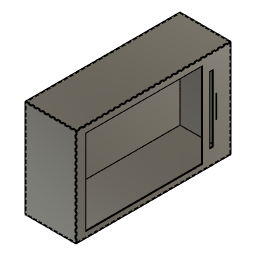
geldautomaat v2 (Autodesk Fusion 360 design; units mm, degrees)
Autodesk Fusion 360 part; units mm, degrees
(part 1 of 3)
sketch "Sketch1" plane through (0, 0, 0) normal (0, 0, 1) x (1, 0, 0)
  line L0 (715.8584, -170.7447) -> (715.8334, -167.7447)
  line L1 (715.8334, -167.7447) -> (707.2277, -167.8174)
  line L2 (707.2277, -167.8174) -> (707.2531, -170.817)
  line L3 (707.2531, -170.817) -> (698.5258, -170.8908)
  line L4 (698.5258, -170.8908) -> (698.5007, -167.8908)
  line L5 (698.5007, -167.8908) -> (689.8951, -167.9631)
  line L6 (689.8951, -167.9631) -> (689.9205, -170.9631)
  line L7 (689.9205, -170.9631) -> (681.1931, -171.0365)
  line L8 (681.1931, -171.0365) -> (681.1677, -168.0365)
  line L9 (681.1677, -168.0365) -> (672.5624, -168.1091)
  line L10 (672.5624, -168.1091) -> (672.5878, -171.1088)
  line L11 (672.5878, -171.1088) -> (663.8601, -171.1825)
  line L12 (663.8601, -171.1825) -> (663.8351, -168.1825)
  line L13 (663.8351, -168.1825) -> (655.2298, -168.2548)
  line L14 (655.2298, -168.2548) -> (655.2552, -171.2548)
  line L15 (655.2552, -171.2548) -> (646.5279, -171.3282)
  line L16 (646.5279, -171.3282) -> (646.5025, -168.3282)
  line L17 (646.5025, -168.3282) -> (637.8972, -168.4005)
  line L18 (637.8972, -168.4005) -> (637.9222, -171.4005)
  line L19 (637.9222, -171.4005) -> (629.1952, -171.4743)
  line L20 (629.1952, -171.4743) -> (629.1702, -168.4743)
  line L21 (629.1702, -168.4743) -> (620.5645, -168.5466)
  line L22 (620.5645, -168.5466) -> (620.5896, -171.5466)
  line L23 (620.5896, -171.5466) -> (611.8626, -171.62)
  line L24 (611.8626, -171.62) -> (611.8372, -168.6199)
  line L25 (611.8372, -168.6199) -> (603.2319, -168.6926)
  line L26 (603.2319, -168.6926) -> (603.257, -171.6923)
  line L27 (603.257, -171.6923) -> (594.5296, -171.7657)
  line L28 (594.5296, -171.7657) -> (594.5046, -168.7664)
  line L29 (594.5046, -168.7664) -> (585.8989, -168.8387)
  line L30 (585.8989, -168.8387) -> (585.9247, -171.8387)
  line L31 (585.9247, -171.8387) -> (577.197, -171.9121)
  line L32 (577.197, -171.9121) -> (577.1719, -168.912)
  line L33 (577.1719, -168.912) -> (568.5663, -168.9844)
  line L34 (568.5663, -168.9844) -> (568.5917, -171.9844)
  line L35 (568.5917, -171.9844) -> (559.8643, -172.0578)
  line L36 (559.8643, -172.0578) -> (559.8389, -169.0581)
  line L37 (559.8389, -169.0581) -> (551.234, -169.1304)
  line L38 (551.234, -169.1304) -> (551.2591, -172.1304)
  line L39 (551.2591, -172.1304) -> (542.5317, -172.2038)
  line L40 (542.5317, -172.2038) -> (542.5063, -169.2038)
  line L41 (542.5063, -169.2038) -> (533.901, -169.2761)
  line L42 (533.901, -169.2761) -> (533.9264, -172.2761)
  line L43 (533.9264, -172.2761) -> (525.1991, -172.3495)
  line L44 (525.1991, -172.3495) -> (525.174, -169.3498)
  line L45 (525.174, -169.3498) -> (516.5684, -169.4222)
  line L46 (516.5684, -169.4222) -> (516.5934, -172.4222)
  line L47 (516.5934, -172.4222) -> (507.8664, -172.4956)
  line L48 (507.8664, -172.4956) -> (507.8414, -169.4955)
  line L49 (507.8414, -169.4955) -> (499.2358, -169.5679)
  line L50 (499.2358, -169.5679) -> (499.2608, -172.5679)
  line L51 (499.2608, -172.5679) -> (490.5338, -172.6413)
  line L52 (490.5338, -172.6413) -> (490.5084, -169.6412)
  line L53 (490.5084, -169.6412) -> (481.9031, -169.7139)
  line L54 (481.9031, -169.7139) -> (481.9285, -172.7136)
  line L55 (481.9285, -172.7136) -> (473.2008, -172.7873)
  line L56 (473.2008, -172.7873) -> (473.1758, -169.7873)
  line L57 (473.1758, -169.7873) -> (464.5705, -169.8596)
  line L58 (464.5705, -169.8596) -> (464.5959, -172.8596)
  line L59 (464.5959, -172.8596) -> (455.8685, -172.933)
  line L60 (455.8685, -172.933) -> (455.8431, -169.933)
  line L61 (455.8431, -169.933) -> (452.8431, -169.9584)
  line L62 (452.8431, -169.9584) -> (452.7782, -162.2135)
  line L63 (452.7782, -162.2135) -> (455.7779, -162.1881)
  line L64 (455.7779, -162.1881) -> (455.7137, -154.5653)
  line L65 (455.7137, -154.5653) -> (452.714, -154.5907)
  line L66 (452.714, -154.5907) -> (452.6487, -146.8459)
  line L67 (452.6487, -146.8459) -> (455.6484, -146.8205)
  line L68 (455.6484, -146.8205) -> (455.5845, -139.1973)
  line L69 (455.5845, -139.1973) -> (452.5845, -139.2227)
  line L70 (452.5845, -139.2227) -> (452.5193, -131.4778)
  line L71 (452.5193, -131.4778) -> (455.5193, -131.4528)
  line L72 (455.5193, -131.4528) -> (455.4551, -123.8296)
  line L73 (455.4551, -123.8296) -> (452.4554, -123.855)
  line L74 (452.4554, -123.855) -> (452.3898, -116.1102)
  line L75 (452.3898, -116.1102) -> (455.3898, -116.0848)
  line L76 (455.3898, -116.0848) -> (455.3256, -108.4616)
  line L77 (455.3256, -108.4616) -> (452.3259, -108.487)
  line L78 (452.3259, -108.487) -> (452.2607, -100.7421)
  line L79 (452.2607, -100.7421) -> (455.2607, -100.7167)
  line L80 (455.2607, -100.7167) -> (455.1961, -93.0943)
  line L81 (455.1961, -93.0943) -> (452.1965, -93.1193)
  line L82 (452.1965, -93.1193) -> (452.1312, -85.3745)
  line L83 (452.1312, -85.3745) -> (455.1312, -85.3494)
  line L84 (455.1312, -85.3494) -> (455.067, -77.7263)
  line L85 (455.067, -77.7263) -> (452.067, -77.7513)
  line L86 (452.067, -77.7513) -> (452.0021, -70.0065)
  line L87 (452.0021, -70.0065) -> (455.0018, -69.9814)
  line L88 (455.0018, -69.9814) -> (454.9376, -62.3583)
  line L89 (454.9376, -62.3583) -> (451.9379, -62.3837)
  line L90 (451.9379, -62.3837) -> (451.8726, -54.6388)
  line L91 (451.8726, -54.6388) -> (454.8723, -54.6137)
  line L92 (454.8723, -54.6137) -> (454.8084, -46.9906)
  line L93 (454.8084, -46.9906) -> (451.8084, -47.0156)
  line L94 (451.8084, -47.0156) -> (451.7432, -39.2708)
  line L95 (451.7432, -39.2708) -> (454.7432, -39.2457)
  line L96 (454.7432, -39.2457) -> (454.679, -31.6229)
  line L97 (454.679, -31.6229) -> (451.6793, -31.648)
  line L98 (451.6793, -31.648) -> (451.614, -23.9031)
  line L99 (451.614, -23.9031) -> (454.6137, -23.8781)
  line L100 (454.6137, -23.8781) -> (454.5887, -20.878)
  line L101 (454.5887, -20.878) -> (463.316, -20.8047)
  line L102 (463.316, -20.8047) -> (463.3411, -23.8043)
  line L103 (463.3411, -23.8043) -> (471.9467, -23.7317)
  line L104 (471.9467, -23.7317) -> (471.9209, -20.732)
  line L105 (471.9209, -20.732) -> (480.6486, -20.6586)
  line L106 (480.6486, -20.6586) -> (480.6737, -23.6583)
  line L107 (480.6737, -23.6583) -> (489.2793, -23.586)
  line L108 (489.2793, -23.586) -> (489.2539, -20.5859)
  line L109 (489.2539, -20.5859) -> (497.9813, -20.5126)
  line L110 (497.9813, -20.5126) -> (498.0067, -23.5122)
  line L111 (498.0067, -23.5122) -> (506.6116, -23.4399)
  line L112 (506.6116, -23.4399) -> (506.5866, -20.4399)
  line L113 (506.5866, -20.4399) -> (515.3136, -20.3665)
  line L114 (515.3136, -20.3665) -> (515.3393, -23.3665)
  line L115 (515.3393, -23.3665) -> (523.9446, -23.2942)
  line L116 (523.9446, -23.2942) -> (523.9192, -20.2942)
  line L117 (523.9192, -20.2942) -> (532.6465, -20.2208)
  line L118 (532.6465, -20.2208) -> (532.6716, -23.2208)
  line L119 (532.6716, -23.2208) -> (541.2772, -23.1482)
  line L120 (541.2772, -23.1482) -> (541.2518, -20.1481)
  line L121 (541.2518, -20.1481) -> (549.9792, -20.0748)
  line L122 (549.9792, -20.0748) -> (550.0042, -23.0748)
  line L123 (550.0042, -23.0748) -> (558.6099, -23.0025)
  line L124 (558.6099, -23.0025) -> (558.5848, -20.0024)
  line L125 (558.5848, -20.0024) -> (567.3118, -19.9291)
  line L126 (567.3118, -19.9291) -> (567.3372, -22.9291)
  line L127 (567.3372, -22.9291) -> (575.9425, -22.8564)
  line L128 (575.9425, -22.8564) -> (575.9171, -19.8568)
  line L129 (575.9171, -19.8568) -> (584.6448, -19.783)
  line L130 (584.6448, -19.783) -> (584.6698, -22.783)
  line L131 (584.6698, -22.783) -> (593.2751, -22.7107)
  line L132 (593.2751, -22.7107) -> (593.2497, -19.7107)
  line L133 (593.2497, -19.7107) -> (601.9771, -19.6373)
  line L134 (601.9771, -19.6373) -> (602.0025, -22.6373)
  line L135 (602.0025, -22.6373) -> (610.6078, -22.5647)
  line L136 (610.6078, -22.5647) -> (610.5827, -19.565)
  line L137 (610.5827, -19.565) -> (619.3097, -19.4913)
  line L138 (619.3097, -19.4913) -> (619.3355, -22.4913)
  line L139 (619.3355, -22.4913) -> (627.9404, -22.419)
  line L140 (627.9404, -22.419) -> (627.9154, -19.419)
  line L141 (627.9154, -19.419) -> (636.6424, -19.3456)
  line L142 (636.6424, -19.3456) -> (636.6678, -22.3456)
  line L143 (636.6678, -22.3456) -> (645.2734, -22.2733)
  line L144 (645.2734, -22.2733) -> (645.248, -19.2733)
  line L145 (645.248, -19.2733) -> (653.9753, -19.1995)
  line L146 (653.9753, -19.1995) -> (654.0004, -22.1995)
  line L147 (654.0004, -22.1995) -> (662.606, -22.1272)
  line L148 (662.606, -22.1272) -> (662.5806, -19.1272)
  line L149 (662.5806, -19.1272) -> (671.308, -19.0538)
  line L150 (671.308, -19.0538) -> (671.333, -22.0538)
  line L151 (671.333, -22.0538) -> (679.9387, -21.9815)
  line L152 (679.9387, -21.9815) -> (679.9133, -18.9815)
  line L153 (679.9133, -18.9815) -> (688.6406, -18.9081)
  line L154 (688.6406, -18.9081) -> (688.666, -21.9078)
  line L155 (688.666, -21.9078) -> (697.2709, -21.8355)
  line L156 (697.2709, -21.8355) -> (697.2459, -18.8355)
  line L157 (697.2459, -18.8355) -> (705.9732, -18.7621)
  line L158 (705.9732, -18.7621) -> (705.9986, -21.7621)
  line L159 (705.9986, -21.7621) -> (714.6039, -21.6894)
  line L160 (714.6039, -21.6894) -> (714.5785, -18.6898)
  line L161 (714.5785, -18.6898) -> (723.3059, -18.6164)
  line L162 (723.3059, -18.6164) -> (723.3313, -21.6157)
  line L163 (723.3313, -21.6157) -> (731.9366, -21.5434)
  line L164 (731.9366, -21.5434) -> (731.9115, -18.5434)
  line L165 (731.9115, -18.5434) -> (740.6385, -18.47)
  line L166 (740.6385, -18.47) -> (740.6639, -21.47)
  line L167 (740.6639, -21.47) -> (743.6636, -21.445)
  line L168 (743.6636, -21.445) -> (743.7288, -29.1898)
  line L169 (743.7288, -29.1898) -> (740.7292, -29.2149)
  line L170 (740.7292, -29.2149) -> (740.7934, -36.838)
  line L171 (740.7934, -36.838) -> (743.7934, -36.813)
  line L172 (743.7934, -36.813) -> (743.8583, -44.5578)
  line L173 (743.8583, -44.5578) -> (740.8583, -44.5829)
  line L174 (740.8583, -44.5829) -> (740.9225, -52.2057)
  line L175 (740.9225, -52.2057) -> (743.9225, -52.1806)
  line L176 (743.9225, -52.1806) -> (743.9874, -59.9252)
  line L177 (743.9874, -59.9252) -> (740.9878, -59.9506)
  line L178 (740.9878, -59.9506) -> (741.052, -67.5737)
  line L179 (741.052, -67.5737) -> (744.052, -67.5487)
  line L180 (744.052, -67.5487) -> (744.1169, -75.2935)
  line L181 (744.1169, -75.2935) -> (741.1172, -75.3186)
  line L182 (741.1172, -75.3186) -> (741.1811, -82.9414)
  line L183 (741.1811, -82.9414) -> (744.1811, -82.9163)
  line L184 (744.1811, -82.9163) -> (744.2464, -90.6612)
  line L185 (744.2464, -90.6612) -> (741.2467, -90.6862)
  line L186 (741.2467, -90.6862) -> (741.3106, -98.3094)
  line L187 (741.3106, -98.3094) -> (744.3106, -98.2843)
  line L188 (744.3106, -98.2843) -> (744.3758, -106.0289)
  line L189 (744.3758, -106.0289) -> (741.3758, -106.0543)
  line L190 (741.3758, -106.0543) -> (741.44, -113.6771)
  line L191 (741.44, -113.6771) -> (744.44, -113.6517)
  line L192 (744.44, -113.6517) -> (744.5049, -121.3969)
  line L193 (744.5049, -121.3969) -> (741.5053, -121.4219)
  line L194 (741.5053, -121.4219) -> (741.5695, -129.0451)
  line L195 (741.5695, -129.0451) -> (744.5692, -129.02)
  line L196 (744.5692, -129.02) -> (744.6344, -136.7645)
  line L197 (744.6344, -136.7645) -> (741.6344, -136.7899)
  line L198 (741.6344, -136.7899) -> (741.6986, -144.4128)
  line L199 (741.6986, -144.4128) -> (744.6986, -144.3877)
  line L200 (744.6986, -144.3877) -> (744.7635, -152.1322)
  line L201 (744.7635, -152.1322) -> (741.7639, -152.1576)
  line L202 (741.7639, -152.1576) -> (741.8281, -159.7808)
  line L203 (741.8281, -159.7808) -> (744.8277, -159.7554)
  line L204 (744.8277, -159.7554) -> (744.8934, -167.5002)
  line L205 (744.8934, -167.5002) -> (741.8933, -167.5256)
  line L206 (741.8933, -167.5256) -> (741.9184, -170.5256)
  line L207 (741.9184, -170.5256) -> (733.191, -170.599)
  line L208 (733.191, -170.599) -> (733.166, -167.5987)
  line L209 (733.166, -167.5987) -> (724.5607, -167.6717)
  line L210 (724.5607, -167.6717) -> (724.5858, -170.6713)
  line L211 (724.5858, -170.6713) -> (715.8584, -170.7447)
  line L212 (300.6837, -267.4691) -> (297.6837, -267.4691)
  line L213 (297.6837, -250.2613) -> (297.6837, -258.9262)
  line L214 (297.6837, -258.9262) -> (300.6837, -258.9262)
  line L215 (300.6837, -250.2613) -> (297.6837, -250.2613)
  line L216 (297.6837, -233.0539) -> (297.6837, -241.7185)
  line L217 (297.6837, -241.7185) -> (300.6837, -241.7185)
  line L218 (300.6837, -233.0539) -> (297.6837, -233.0539)
  line L219 (297.6837, -215.8465) -> (297.6837, -224.5111)
  line L220 (297.6837, -224.5111) -> (300.6837, -224.5111)
  line L221 (300.6837, -215.8465) -> (297.6837, -215.8465)
  line L222 (297.6837, -198.6388) -> (297.6837, -207.3037)
  line L223 (297.6837, -207.3037) -> (300.6837, -207.3037)
  line L224 (300.6837, -198.6388) -> (297.6837, -198.6388)
  line L225 (297.6837, -190.0959) -> (297.6837, -181.431)
  line L226 (297.6837, -190.0959) -> (300.6837, -190.0959)
  line L227 (297.6837, -181.4314) -> (297.6837, -178.4314)
  line L228 (297.6837, -178.4314) -> (300.6837, -178.4314)
  line L229 (308.3679, -181.4314) -> (300.6837, -181.4314)
  line L230 (300.6837, -258.9262) -> (300.6837, -267.4691)
  line L231 (300.6837, -241.7185) -> (300.6837, -250.2613)
  line L232 (300.6837, -224.5111) -> (300.6837, -233.0539)
  line L233 (300.6837, -207.3037) -> (300.6837, -215.8465)
  line L234 (300.6837, -190.0959) -> (300.6837, -198.6388)
  line L235 (300.6837, -178.4314) -> (300.7448, -178.4314)
  line L236 (300.7448, -178.4314) -> (300.7448, -181.4314)
  line L237 (308.3679, -178.4314) -> (308.3679, -181.4314)
  line L238 (316.1131, -178.4314) -> (308.3679, -178.4314)
  line L239 (316.1131, -181.4314) -> (316.1131, -178.4314)
  line L240 (323.7363, -181.4314) -> (316.1131, -181.4314)
  line L241 (323.7363, -178.4314) -> (323.7363, -181.4314)
  line L242 (331.4815, -178.4314) -> (323.7363, -178.4314)
  line L243 (331.4815, -181.4314) -> (331.4815, -178.4314)
  line L244 (339.1047, -181.4314) -> (331.4815, -181.4314)
  line L245 (339.1047, -178.4314) -> (339.1047, -181.4314)
  line L246 (346.8499, -178.4314) -> (339.1047, -178.4314)
  line L247 (346.8499, -181.4314) -> (346.8499, -178.4314)
  line L248 (354.473, -181.4314) -> (346.8499, -181.4314)
  line L249 (354.473, -178.4314) -> (354.473, -181.4314)
  line L250 (362.2183, -178.4314) -> (354.473, -178.4314)
  line L251 (362.2183, -181.4314) -> (362.2183, -178.4314)
  line L252 (369.8414, -181.4314) -> (362.2183, -181.4314)
  line L253 (369.8414, -178.4314) -> (369.8414, -181.4314)
  line L254 (377.5866, -178.4314) -> (369.8414, -178.4314)
  line L255 (377.5866, -181.4314) -> (377.5866, -178.4314)
  line L256 (385.2101, -181.4314) -> (377.5866, -181.4314)
  line L257 (385.2101, -178.4314) -> (385.2101, -181.4314)
  line L258 (392.955, -178.4314) -> (385.2101, -178.4314)
  line L259 (392.955, -181.4314) -> (392.955, -178.4314)
  line L260 (400.5782, -181.4314) -> (392.955, -181.4314)
  line L261 (400.5782, -178.4314) -> (400.5782, -181.4314)
  line L262 (408.3234, -178.4314) -> (400.5782, -178.4314)
  line L263 (408.3234, -181.4314) -> (408.3234, -178.4314)
  line L264 (415.9465, -181.4314) -> (408.3234, -181.4314)
  line L265 (415.9465, -178.4314) -> (415.9465, -181.4314)
  line L266 (423.6921, -178.4314) -> (415.9465, -178.4314)
  line L267 (423.6921, -181.4314) -> (423.6921, -178.4314)
  line L268 (431.3149, -181.4314) -> (423.6921, -181.4314)
  line L269 (431.3149, -178.4314) -> (431.3149, -181.4314)
  line L270 (439.0601, -178.4314) -> (431.3149, -178.4314)
  line L271 (439.0601, -181.4314) -> (439.0601, -178.4314)
  line L272 (446.7443, -181.4314) -> (439.0601, -181.4314)
  line L273 (446.6833, -178.4314) -> (446.6833, -181.4314)
  line L274 (446.6833, -178.4314) -> (446.7443, -178.4314)
  line L275 (446.7443, -267.4691) -> (446.7443, -258.9259)
  line L276 (449.7443, -267.4691) -> (446.7443, -267.4691)
  line L277 (446.7443, -258.9262) -> (449.7443, -258.9262)
  line L278 (446.7443, -250.2613) -> (446.7443, -241.7185)
  line L279 (449.7443, -250.2613) -> (446.7443, -250.2613)
  line L280 (446.7443, -241.7185) -> (449.7443, -241.7185)
  line L281 (446.7443, -233.0539) -> (446.7443, -224.5111)
  line L282 (449.7443, -233.0539) -> (446.7443, -233.0539)
  line L283 (446.7443, -224.5111) -> (449.7443, -224.5111)
  line L284 (446.7443, -215.8465) -> (446.7443, -207.3033)
  line L285 (449.7443, -215.8465) -> (446.7443, -215.8465)
  line L286 (446.7443, -207.3037) -> (449.7443, -207.3037)
  line L287 (446.7443, -198.6388) -> (446.7443, -190.0959)
  line L288 (449.7443, -198.6388) -> (446.7443, -198.6388)
  line L289 (446.7443, -190.0959) -> (449.7443, -190.0959)
  line L290 (446.7443, -178.4314) -> (449.7443, -178.4314)
  line L291 (449.7443, -267.4687) -> (449.7443, -276.1336)
  line L292 (449.7443, -276.1336) -> (446.7443, -276.1336)
  line L293 (446.7443, -276.1336) -> (446.7443, -284.6765)
  line L294 (446.7443, -284.6765) -> (449.7443, -284.6761)
  line L295 (449.7443, -284.6761) -> (449.7443, -293.3414)
  line L296 (449.7443, -293.3414) -> (446.7443, -293.341)
  line L297 (446.7443, -293.341) -> (446.7443, -301.8839)
  line L298 (446.7443, -301.8839) -> (449.7443, -301.8839)
  line L299 (449.7443, -301.8839) -> (449.7443, -310.5488)
  line L300 (449.7443, -310.5488) -> (446.7443, -310.5484)
  line L301 (446.7443, -310.5484) -> (446.7443, -319.0916)
  line L302 (446.7443, -319.0916) -> (449.7443, -319.0913)
  line L303 (449.7443, -319.0913) -> (449.7443, -327.7562)
  line L304 (449.7443, -327.7562) -> (446.7443, -327.7562)
  line L305 (446.7443, -327.7562) -> (446.7443, -336.299)
  line L306 (446.7443, -336.299) -> (449.7443, -336.299)
  line L307 (449.7443, -336.299) -> (449.7443, -344.9639)
  line L308 (449.7443, -344.9639) -> (446.7443, -344.9636)
  line L309 (446.7443, -344.9636) -> (446.7443, -353.5064)
  line L310 (446.7443, -353.5064) -> (449.7443, -353.5064)
  line L311 (449.7443, -353.5064) -> (449.7443, -362.1713)
  line L312 (449.7443, -362.1713) -> (446.7443, -362.171)
  line L313 (446.7443, -362.171) -> (446.7443, -370.7142)
  line L314 (446.7443, -370.7142) -> (449.7443, -370.7138)
  line L315 (449.7443, -370.7138) -> (449.7443, -379.3784)
  line L316 (449.7443, -379.3784) -> (446.7443, -379.3784)
  line L317 (446.7443, -379.3784) -> (446.7443, -387.9216)
  line L318 (446.7443, -387.9216) -> (449.7443, -387.9216)
  line L319 (449.7443, -387.9216) -> (449.7443, -396.5861)
  line L320 (449.7443, -396.5861) -> (446.7443, -396.5858)
  line L321 (446.7443, -396.5858) -> (446.7443, -405.129)
  line L322 (446.7443, -405.129) -> (449.7443, -405.129)
  line L323 (449.7443, -405.129) -> (449.7443, -413.7935)
  line L324 (449.7443, -413.7935) -> (446.7443, -413.7935)
  line L325 (446.7443, -413.7935) -> (446.7443, -422.3367)
  line L326 (446.7443, -422.3367) -> (449.7443, -422.3364)
  line L327 (449.7443, -422.3364) -> (449.7443, -431.0009)
  line L328 (449.7443, -431.0009) -> (446.7443, -431.0009)
  line L329 (446.7443, -431.0009) -> (446.7443, -439.5441)
  line L330 (446.7443, -439.5441) -> (449.7443, -439.5438)
  line L331 (449.7443, -439.5438) -> (449.7443, -448.2087)
  line L332 (449.7443, -448.2087) -> (446.7443, -448.2087)
  line L333 (446.7443, -448.2087) -> (446.7443, -456.7515)
  line L334 (446.7443, -456.7515) -> (449.7443, -456.7512)
  line L335 (449.7443, -456.7512) -> (449.7443, -465.4161)
  line L336 (449.7443, -465.4161) -> (446.7443, -465.4161)
  line L337 (446.7443, -465.4161) -> (446.7443, -473.9589)
  line L338 (446.7443, -473.9589) -> (449.7443, -473.9586)
  line L339 (449.7443, -473.9586) -> (449.7443, -482.6235)
  line L340 (449.7443, -482.6235) -> (446.7443, -482.6235)
  line L341 (446.7443, -482.6235) -> (446.7443, -491.1663)
  line L342 (446.7443, -491.1663) -> (449.7443, -491.166)
  line L343 (449.7443, -491.166) -> (449.7443, -499.8312)
  line L344 (449.7443, -499.8312) -> (446.7443, -499.8312)
  line L345 (446.7443, -499.8312) -> (446.7443, -508.3737)
  line L346 (446.7443, -508.3737) -> (449.7443, -508.3737)
  line L347 (449.7443, -508.3737) -> (449.7443, -517.0386)
  line L348 (449.7443, -517.0386) -> (446.7443, -517.0386)
  line L349 (446.7443, -517.0386) -> (446.7443, -525.5815)
  line L350 (446.7443, -525.5815) -> (449.7443, -525.5811)
  line L351 (449.7443, -525.5811) -> (449.7443, -534.246)
  line L352 (449.7443, -534.246) -> (446.7443, -534.246)
  line L353 (446.7443, -534.246) -> (446.7443, -542.7889)
  line L354 (446.7443, -542.7889) -> (449.7443, -542.7885)
  line L355 (449.7443, -542.7885) -> (449.7443, -551.4538)
  line L356 (449.7443, -551.4538) -> (446.7443, -551.4538)
  line L357 (446.7443, -551.4538) -> (446.7443, -559.9966)
  line L358 (446.7443, -559.9966) -> (449.7443, -559.9963)
  line L359 (449.7443, -559.9963) -> (449.7443, -568.6612)
  line L360 (449.7443, -568.6612) -> (446.7443, -568.6612)
  line L361 (446.7443, -568.6612) -> (446.7443, -577.204)
  line L362 (446.7443, -577.204) -> (449.7443, -577.2037)
  line L363 (449.7443, -577.2037) -> (449.7443, -585.8686)
  line L364 (449.7443, -585.8686) -> (446.7443, -585.8686)
  line L365 (446.7443, -585.8686) -> (446.7443, -594.4114)
  line L366 (446.7443, -594.4114) -> (449.7443, -594.4111)
  line L367 (449.7443, -594.4111) -> (449.7443, -603.0763)
  line L368 (449.7443, -603.0763) -> (446.7443, -603.0763)
  line L369 (446.7443, -603.0763) -> (446.7443, -611.6192)
  line L370 (446.7443, -611.6192) -> (449.7443, -611.6188)
  line L371 (449.7443, -611.6188) -> (449.7443, -620.2837)
  line L372 (449.7443, -620.2837) -> (446.7443, -620.2837)
  line L373 (446.7443, -620.2837) -> (446.7443, -628.8266)
  line L374 (446.7443, -628.8266) -> (449.7443, -628.8266)
  line L375 (449.7443, -628.8266) -> (449.7443, -637.4911)
  line L376 (449.7443, -637.4911) -> (449.7443, -640.4911)
  line L377 (449.7443, -640.4911) -> (446.7443, -640.4911)
  line L378 (446.7443, -640.4911) -> (446.6833, -640.4911)
  line L379 (446.6833, -640.4911) -> (446.6833, -637.4911)
  line L380 (446.6833, -637.4911) -> (446.7443, -637.4911)
  line L381 (446.7443, -637.4911) -> (439.0601, -637.4911)
  line L382 (439.0601, -637.4911) -> (439.0601, -640.4911)
  line L383 (439.0601, -640.4911) -> (431.3149, -640.4911)
  line L384 (431.3149, -640.4911) -> (431.3146, -637.4911)
  line L385 (431.3146, -637.4911) -> (423.6921, -637.4911)
  line L386 (423.6921, -637.4911) -> (423.6921, -640.4911)
  line L387 (423.6921, -640.4911) -> (415.9465, -640.4911)
  line L388 (415.9465, -640.4911) -> (415.9465, -637.4911)
  line L389 (415.9465, -637.4911) -> (408.3234, -637.4911)
  line L390 (408.3234, -637.4911) -> (408.3234, -640.4911)
  line L391 (408.3234, -640.4911) -> (400.5782, -640.4911)
  line L392 (400.5782, -640.4911) -> (400.5782, -637.4911)
  line L393 (400.5782, -637.4911) -> (392.955, -637.4911)
  line L394 (392.955, -637.4911) -> (392.955, -640.4911)
  line L395 (392.955, -640.4911) -> (385.2101, -640.4911)
  line L396 (385.2101, -640.4911) -> (385.2098, -637.4911)
  line L397 (385.2098, -637.4911) -> (377.5866, -637.4911)
  line L398 (377.5866, -637.4911) -> (377.5866, -640.4911)
  line L399 (377.5866, -640.4911) -> (369.8414, -640.4911)
  line L400 (369.8414, -640.4911) -> (369.8414, -637.4911)
  line L401 (369.8414, -637.4911) -> (362.2183, -637.4911)
  line L402 (362.2183, -637.4911) -> (362.2183, -640.4911)
  line L403 (362.2183, -640.4911) -> (354.473, -640.4911)
  line L404 (354.473, -640.4911) -> (354.473, -637.4911)
  line L405 (354.473, -637.4911) -> (346.8499, -637.4911)
  line L406 (346.8499, -637.4911) -> (346.8499, -640.4911)
  line L407 (346.8499, -640.4911) -> (339.1047, -640.4911)
  line L408 (339.1047, -640.4911) -> (339.1047, -637.4911)
  line L409 (339.1047, -637.4911) -> (331.4815, -637.4911)
  line L410 (331.4815, -637.4911) -> (331.4815, -640.4911)
  line L411 (331.4815, -640.4911) -> (323.7363, -640.4911)
  line L412 (323.7363, -640.4911) -> (323.7363, -637.4911)
  line L413 (323.7363, -637.4911) -> (316.1131, -637.4911)
  line L414 (316.1131, -637.4911) -> (316.1131, -640.4911)
  line L415 (316.1131, -640.4911) -> (308.3679, -640.4911)
  line L416 (308.3679, -640.4911) -> (308.3679, -637.4911)
  line L417 (308.3679, -637.4911) -> (300.6837, -637.4911)
  line L418 (300.6837, -637.4911) -> (300.7448, -637.4911)
  line L419 (300.7448, -637.4911) -> (300.7448, -640.4911)
  line L420 (300.7448, -640.4911) -> (300.6837, -640.4911)
  line L421 (300.6837, -640.4911) -> (297.6837, -640.4911)
  line L422 (297.6837, -640.4911) -> (297.6837, -637.4908)
  line L423 (297.6837, -637.4908) -> (297.6837, -628.8266)
  line L424 (297.6837, -628.8266) -> (300.6837, -628.8266)
  line L425 (300.6837, -628.8266) -> (300.6837, -620.2837)
  line L426 (300.6837, -620.2837) -> (297.6837, -620.2837)
  line L427 (297.6837, -620.2837) -> (297.6837, -611.6192)
  line L428 (297.6837, -611.6192) -> (300.6837, -611.6192)
  line L429 (300.6837, -611.6192) -> (300.6837, -603.0763)
  line L430 (300.6837, -603.0763) -> (297.6837, -603.0763)
  line L431 (297.6837, -603.0763) -> (297.6837, -594.4114)
  line L432 (297.6837, -594.4114) -> (300.6837, -594.4114)
  line L433 (300.6837, -594.4114) -> (300.6837, -585.8686)
  line L434 (300.6837, -585.8686) -> (297.6837, -585.8686)
  line L435 (297.6837, -585.8686) -> (297.6837, -577.204)
  line L436 (297.6837, -577.204) -> (300.6837, -577.204)
  line L437 (300.6837, -577.204) -> (300.6837, -568.6612)
  line L438 (300.6837, -568.6612) -> (297.6837, -568.6612)
  line L439 (297.6837, -568.6612) -> (297.6837, -559.9966)
  line L440 (297.6837, -559.9966) -> (300.6837, -559.9966)
  line L441 (300.6837, -559.9966) -> (300.6837, -551.4538)
  line L442 (300.6837, -551.4538) -> (297.6837, -551.4538)
  line L443 (297.6837, -551.4538) -> (297.6837, -542.7889)
  line L444 (297.6837, -542.7889) -> (300.6837, -542.7889)
  line L445 (300.6837, -542.7889) -> (300.6837, -534.246)
  line L446 (300.6837, -534.246) -> (297.6837, -534.246)
  line L447 (297.6837, -534.246) -> (297.6837, -525.5815)
  line L448 (297.6837, -525.5815) -> (300.6837, -525.5815)
  line L449 (300.6837, -525.5815) -> (300.6837, -517.0386)
  line L450 (300.6837, -517.0386) -> (297.6837, -517.0386)
  line L451 (297.6837, -517.0386) -> (297.6837, -508.3737)
  line L452 (297.6837, -508.3737) -> (300.6837, -508.3737)
  line L453 (300.6837, -508.3737) -> (300.6837, -499.8312)
  line L454 (300.6837, -499.8312) -> (297.6837, -499.8312)
  line L455 (297.6837, -499.8312) -> (297.6837, -491.1663)
  line L456 (297.6837, -491.1663) -> (300.6837, -491.1663)
  line L457 (300.6837, -491.1663) -> (300.6837, -482.6235)
  line L458 (300.6837, -482.6235) -> (297.6837, -482.6235)
  line L459 (297.6837, -482.6235) -> (297.6837, -473.9589)
  line L460 (297.6837, -473.9589) -> (300.6837, -473.9589)
  line L461 (300.6837, -473.9589) -> (300.6837, -465.4161)
  line L462 (300.6837, -465.4161) -> (297.6837, -465.4161)
  line L463 (297.6837, -465.4161) -> (297.6837, -456.7515)
  line L464 (297.6837, -456.7515) -> (300.6837, -456.7515)
  line L465 (300.6837, -456.7515) -> (300.6837, -448.2087)
  line L466 (300.6837, -448.2087) -> (297.6837, -448.2087)
  line L467 (297.6837, -448.2087) -> (297.6837, -439.5441)
  line L468 (297.6837, -439.5441) -> (300.6837, -439.5441)
  line L469 (300.6837, -439.5441) -> (300.6837, -431.0009)
  line L470 (300.6837, -431.0009) -> (297.6837, -431.0009)
  line L471 (297.6837, -431.0009) -> (297.6837, -422.3367)
  line L472 (297.6837, -422.3367) -> (300.6837, -422.3367)
  line L473 (300.6837, -422.3367) -> (300.6837, -413.7935)
  line L474 (300.6837, -413.7935) -> (297.6837, -413.7935)
  line L475 (297.6837, -413.7935) -> (297.6837, -405.129)
  line L476 (297.6837, -405.129) -> (300.6837, -405.129)
  line L477 (300.6837, -405.129) -> (300.6837, -396.5861)
  line L478 (300.6837, -396.5861) -> (297.6837, -396.5861)
  line L479 (297.6837, -396.5861) -> (297.6837, -387.9216)
  line L480 (297.6837, -387.9216) -> (300.6837, -387.9216)
  line L481 (300.6837, -387.9216) -> (300.6837, -379.3784)
  line L482 (300.6837, -379.3784) -> (297.6837, -379.3784)
  line L483 (297.6837, -379.3784) -> (297.6837, -370.7142)
  line L484 (297.6837, -370.7142) -> (300.6837, -370.7142)
  line L485 (300.6837, -370.7142) -> (300.6837, -362.1713)
  line L486 (300.6837, -362.1713) -> (297.6837, -362.1713)
  line L487 (297.6837, -362.1713) -> (297.6837, -353.5064)
  line L488 (297.6837, -353.5064) -> (300.6837, -353.5064)
  line L489 (300.6837, -353.5064) -> (300.6837, -344.9639)
  line L490 (300.6837, -344.9639) -> (297.6837, -344.9639)
  line L491 (297.6837, -344.9639) -> (297.6837, -336.299)
  line L492 (297.6837, -336.299) -> (300.6837, -336.299)
  line L493 (300.6837, -336.299) -> (300.6837, -327.7562)
  line L494 (300.6837, -327.7562) -> (297.6837, -327.7562)
  line L495 (297.6837, -327.7562) -> (297.6837, -319.0916)
  line L496 (297.6837, -319.0916) -> (300.6837, -319.0916)
  line L497 (300.6837, -319.0916) -> (300.6837, -310.5488)
  line L498 (300.6837, -310.5488) -> (297.6837, -310.5488)
  line L499 (297.6837, -310.5488) -> (297.6837, -301.8839)
  line L500 (297.6837, -301.8839) -> (300.6837, -301.8839)
  line L501 (300.6837, -301.8839) -> (300.6837, -293.3414)
  line L502 (300.6837, -293.3414) -> (297.6837, -293.3414)
  line L503 (297.6837, -293.3414) -> (297.6837, -284.6765)
  line L504 (297.6837, -284.6765) -> (300.6837, -284.6765)
  line L505 (300.6837, -284.6765) -> (300.6837, -276.1336)
  line L506 (300.6837, -276.1336) -> (297.6837, -276.1336)
  line L507 (297.6837, -276.1336) -> (297.6837, -267.4691)
  line L508 (449.7443, -258.9262) -> (449.7443, -250.2613)
  line L509 (449.7443, -241.7185) -> (449.7443, -233.0536)
  line L510 (449.7443, -224.5111) -> (449.7443, -215.8462)
  line L511 (449.7443, -207.3037) -> (449.7443, -198.6388)
  line L512 (449.7443, -190.0959) -> (449.7443, -181.431)
  line L513 (449.7443, -181.4314) -> (449.7443, -178.4314)
  line L514 (273.7669, -170.1263) -> (273.7573, -167.1263)
  line L515 (273.7573, -167.1263) -> (265.1521, -167.1535)
  line L516 (265.1521, -167.1535) -> (265.1616, -170.1538)
  line L517 (265.1616, -170.1538) -> (256.4339, -170.1813)
  line L518 (256.4339, -170.1813) -> (256.4244, -167.1813)
  line L519 (256.4244, -167.1813) -> (247.8187, -167.2088)
  line L520 (247.8187, -167.2088) -> (247.8282, -170.2089)
  line L521 (247.8282, -170.2089) -> (239.1009, -170.2371)
  line L522 (239.1009, -170.2371) -> (239.091, -167.2371)
  line L523 (239.091, -167.2371) -> (230.4854, -167.2646)
  line L524 (230.4854, -167.2646) -> (230.4953, -170.2646)
  line L525 (230.4953, -170.2646) -> (221.7676, -170.2925)
  line L526 (221.7676, -170.2925) -> (221.7577, -167.2924)
  line L527 (221.7577, -167.2924) -> (213.1524, -167.32)
  line L528 (213.1524, -167.32) -> (213.1619, -170.32)
  line L529 (213.1619, -170.32) -> (204.4342, -170.3478)
  line L530 (204.4342, -170.3478) -> (204.4247, -167.3478)
  line L531 (204.4247, -167.3478) -> (195.819, -167.375)
  line L532 (195.819, -167.375) -> (195.8286, -170.375)
  line L533 (195.8286, -170.375) -> (187.1012, -170.4029)
  line L534 (187.1012, -170.4029) -> (187.0913, -167.4029)
  line L535 (187.0913, -167.4029) -> (178.4857, -167.4304)
  line L536 (178.4857, -167.4304) -> (178.4956, -170.4304)
  line L537 (178.4956, -170.4304) -> (169.7679, -170.4583)
  line L538 (169.7679, -170.4583) -> (169.7584, -167.4586)
  line L539 (169.7584, -167.4586) -> (161.1527, -167.4861)
  line L540 (161.1527, -167.4861) -> (161.1622, -170.4861)
  line L541 (161.1622, -170.4861) -> (152.4349, -170.514)
  line L542 (152.4349, -170.514) -> (152.425, -167.514)
  line L543 (152.425, -167.514) -> (143.8194, -167.5412)
  line L544 (143.8194, -167.5412) -> (143.8293, -170.5415)
  line L545 (143.8293, -170.5415) -> (135.1016, -170.569)
  line L546 (135.1016, -170.569) -> (135.0917, -167.569)
  line L547 (135.0917, -167.569) -> (126.4864, -167.5965)
  line L548 (126.4864, -167.5965) -> (126.4959, -170.5966)
  line L549 (126.4959, -170.5966) -> (117.7686, -170.6244)
  line L550 (117.7686, -170.6244) -> (117.7587, -167.6244)
  line L551 (117.7587, -167.6244) -> (109.1531, -167.6519)
  line L552 (109.1531, -167.6519) -> (109.1626, -170.6519)
  line L553 (109.1626, -170.6519) -> (100.4352, -170.6798)
  line L554 (100.4352, -170.6798) -> (100.4254, -167.6798)
  line L555 (100.4254, -167.6798) -> (91.8197, -167.7077)
  line L556 (91.8197, -167.7077) -> (91.8296, -170.7073)
  line L557 (91.8296, -170.7073) -> (83.1019, -170.7356)
  line L558 (83.1019, -170.7356) -> (83.0924, -167.7355)
  line L559 (83.0924, -167.7355) -> (74.4867, -167.7627)
  line L560 (74.4867, -167.7627) -> (74.4962, -170.7627)
  line L561 (74.4962, -170.7627) -> (65.7689, -170.7906)
  line L562 (65.7689, -170.7906) -> (65.759, -167.7906)
  line L563 (65.759, -167.7906) -> (57.1534, -167.8181)
  line L564 (57.1534, -167.8181) -> (57.1629, -170.8181)
  line L565 (57.1629, -170.8181) -> (48.4356, -170.846)
  line L566 (48.4356, -170.846) -> (48.426, -167.846)
  line L567 (48.426, -167.846) -> (39.82, -167.8735)
  line L568 (39.82, -167.8735) -> (39.8299, -170.8735)
  line L569 (39.8299, -170.8735) -> (31.1022, -170.9014)
  line L570 (31.1022, -170.9014) -> (31.0927, -167.9013)
  line L571 (31.0927, -167.9013) -> (22.4871, -167.9289)
  line L572 (22.4871, -167.9289) -> (22.4966, -170.9289)
  line L573 (22.4966, -170.9289) -> (13.7692, -170.9567)
  line L574 (13.7692, -170.9567) -> (13.7594, -167.9567)
  line L575 (13.7594, -167.9567) -> (10.7597, -167.9663)
  line L576 (10.7597, -167.9663) -> (10.7346, -160.2214)
  line L577 (10.7346, -160.2214) -> (13.7347, -160.2119)
  line L578 (13.7347, -160.2119) -> (13.7103, -152.5884)
  line L579 (13.7103, -152.5884) -> (10.7103, -152.5982)
  line L580 (10.7103, -152.5982) -> (10.6856, -144.8527)
  line L581 (10.6856, -144.8527) -> (13.6856, -144.8431)
  line L582 (13.6856, -144.8431) -> (13.6613, -137.2203)
  line L583 (13.6613, -137.2203) -> (10.6613, -137.2295)
  line L584 (10.6613, -137.2295) -> (10.6366, -129.4846)
  line L585 (10.6366, -129.4846) -> (13.6366, -129.4751)
  line L586 (13.6366, -129.4751) -> (13.6122, -121.8516)
  line L587 (13.6122, -121.8516) -> (10.6122, -121.8615)
  line L588 (10.6122, -121.8615) -> (10.5875, -114.1159)
  line L589 (10.5875, -114.1159) -> (13.5876, -114.1067)
  line L590 (13.5876, -114.1067) -> (13.5632, -106.4836)
  line L591 (13.5632, -106.4836) -> (10.5632, -106.4931)
  line L592 (10.5632, -106.4931) -> (10.5385, -98.7479)
  line L593 (10.5385, -98.7479) -> (13.5382, -98.7384)
  line L594 (13.5382, -98.7384) -> (13.5142, -91.1152)
  line L595 (13.5142, -91.1152) -> (10.5142, -91.1251)
  line L596 (10.5142, -91.1251) -> (10.4895, -83.3799)
  line L597 (10.4895, -83.3799) -> (13.4891, -83.37)
  line L598 (13.4891, -83.37) -> (13.4648, -75.7468)
  line L599 (13.4648, -75.7468) -> (10.4651, -75.7564)
  line L600 (10.4651, -75.7564) -> (10.4404, -68.0115)
  line L601 (10.4404, -68.0115) -> (13.4401, -68.002)
  line L602 (13.4401, -68.002) -> (13.4158, -60.3785)
  line L603 (13.4158, -60.3785) -> (10.4157, -60.3883)
  line L604 (10.4157, -60.3883) -> (10.3914, -52.6431)
  line L605 (10.3914, -52.6431) -> (13.3911, -52.6333)
  line L606 (13.3911, -52.6333) -> (13.3667, -45.0105)
  line L607 (13.3667, -45.0105) -> (10.3667, -45.0196)
  line L608 (10.3667, -45.0196) -> (10.342, -37.2748)
  line L609 (10.342, -37.2748) -> (13.342, -37.2652)
  line L610 (13.342, -37.2652) -> (13.3177, -29.6417)
  line L611 (13.3177, -29.6417) -> (10.3177, -29.6516)
  line L612 (10.3177, -29.6516) -> (10.293, -21.9067)
  line L613 (10.293, -21.9067) -> (13.293, -21.8969)
  line L614 (13.293, -21.8969) -> (13.2835, -18.8968)
  line L615 (13.2835, -18.8968) -> (22.0112, -18.869)
  line L616 (22.0112, -18.869) -> (22.0203, -21.869)
  line L617 (22.0203, -21.869) -> (30.626, -21.8415)
  line L618 (30.626, -21.8415) -> (30.6164, -18.8415)
  line L619 (30.6164, -18.8415) -> (39.3441, -18.8136)
  line L620 (39.3441, -18.8136) -> (39.3537, -21.8136)
  line L621 (39.3537, -21.8136) -> (47.9593, -21.7861)
  line L622 (47.9593, -21.7861) -> (47.9498, -18.7861)
  line L623 (47.9498, -18.7861) -> (56.6775, -18.7582)
  line L624 (56.6775, -18.7582) -> (56.687, -21.7582)
  line L625 (56.687, -21.7582) -> (65.2927, -21.7311)
  line L626 (65.2927, -21.7311) -> (65.2831, -18.731)
  line L627 (65.2831, -18.731) -> (74.0105, -18.7032)
  line L628 (74.0105, -18.7032) -> (74.02, -21.7032)
  line L629 (74.02, -21.7032) -> (82.6256, -21.6753)
  line L630 (82.6256, -21.6753) -> (82.6161, -18.6753)
  line L631 (82.6161, -18.6753) -> (91.3438, -18.6474)
  line L632 (91.3438, -18.6474) -> (91.3533, -21.6474)
  line L633 (91.3533, -21.6474) -> (99.959, -21.6199)
  line L634 (99.959, -21.6199) -> (99.9495, -18.6199)
  line L635 (99.9495, -18.6199) -> (108.6772, -18.592)
  line L636 (108.6772, -18.592) -> (108.6863, -21.5921)
  line L637 (108.6863, -21.5921) -> (117.292, -21.5645)
  line L638 (117.292, -21.5645) -> (117.2828, -18.5645)
  line L639 (117.2828, -18.5645) -> (126.0101, -18.5367)
  line L640 (126.0101, -18.5367) -> (126.0197, -21.537)
  line L641 (126.0197, -21.537) -> (134.6253, -21.5095)
  line L642 (134.6253, -21.5095) -> (134.6158, -18.5095)
  line L643 (134.6158, -18.5095) -> (143.3435, -18.4816)
  line L644 (143.3435, -18.4816) -> (143.353, -21.4816)
  line L645 (143.353, -21.4816) -> (151.9586, -21.4538)
  line L646 (151.9586, -21.4538) -> (151.9491, -18.4541)
  line L647 (151.9491, -18.4541) -> (160.6765, -18.4259)
  line L648 (160.6765, -18.4259) -> (160.686, -21.4259)
  line L649 (160.686, -21.4259) -> (169.2916, -21.3984)
  line L650 (169.2916, -21.3984) -> (169.2821, -18.3984)
  line L651 (169.2821, -18.3984) -> (178.0098, -18.3705)
  line L652 (178.0098, -18.3705) -> (178.0193, -21.3705)
  line L653 (178.0193, -21.3705) -> (186.625, -21.3434)
  line L654 (186.625, -21.3434) -> (186.6155, -18.3433)
  line L655 (186.6155, -18.3433) -> (195.3428, -18.3155)
  line L656 (195.3428, -18.3155) -> (195.3527, -21.3155)
  line L657 (195.3527, -21.3155) -> (203.958, -21.288)
  line L658 (203.958, -21.288) -> (203.9488, -18.288)
  line L659 (203.9488, -18.288) -> (212.6761, -18.2601)
  line L660 (212.6761, -18.2601) -> (212.6857, -21.2601)
  line L661 (212.6857, -21.2601) -> (221.2913, -21.2326)
  line L662 (221.2913, -21.2326) -> (221.2818, -18.2326)
  line L663 (221.2818, -18.2326) -> (230.0095, -18.2047)
  line L664 (230.0095, -18.2047) -> (230.019, -21.2044)
  line L665 (230.019, -21.2044) -> (238.6246, -21.1772)
  line L666 (238.6246, -21.1772) -> (238.6151, -18.1768)
  line L667 (238.6151, -18.1768) -> (247.3425, -18.1493)
  line L668 (247.3425, -18.1493) -> (247.3523, -21.1493)
  line L669 (247.3523, -21.1493) -> (255.9576, -21.1218)
  line L670 (255.9576, -21.1218) -> (255.9481, -18.1218)
  line L671 (255.9481, -18.1218) -> (264.6758, -18.0939)
  line L672 (264.6758, -18.0939) -> (264.6853, -21.0939)
  line L673 (264.6853, -21.0939) -> (273.291, -21.0664)
  line L674 (273.291, -21.0664) -> (273.2814, -18.0664)
  line L675 (273.2814, -18.0664) -> (282.0088, -18.0385)
  line L676 (282.0088, -18.0385) -> (282.0187, -21.0386)
  line L677 (282.0187, -21.0386) -> (290.624, -21.011)
  line L678 (290.624, -21.011) -> (290.6148, -18.011)
  line L679 (290.6148, -18.011) -> (299.3421, -17.9832)
  line L680 (299.3421, -17.9832) -> (299.3517, -20.9828)
  line L681 (299.3517, -20.9828) -> (302.3517, -20.9736)
  line L682 (302.3517, -20.9736) -> (302.3764, -28.7185)
  line L683 (302.3764, -28.7185) -> (299.3764, -28.7284)
  line L684 (299.3764, -28.7284) -> (299.4007, -36.3515)
  line L685 (299.4007, -36.3515) -> (302.4007, -36.342)
  line L686 (302.4007, -36.342) -> (302.4254, -44.0872)
  line L687 (302.4254, -44.0872) -> (299.4257, -44.0964)
  line L688 (299.4257, -44.0964) -> (299.4497, -51.7196)
  line L689 (299.4497, -51.7196) -> (302.4497, -51.71)
  line L690 (302.4497, -51.71) -> (302.4748, -59.4553)
  line L691 (302.4748, -59.4553) -> (299.4748, -59.4651)
  line L692 (299.4748, -59.4651) -> (299.4991, -67.0879)
  line L693 (299.4991, -67.0879) -> (302.4988, -67.0788)
  line L694 (302.4988, -67.0788) -> (302.5238, -74.8236)
  line L695 (302.5238, -74.8236) -> (299.5238, -74.8332)
  line L696 (299.5238, -74.8332) -> (299.5482, -82.4563)
  line L697 (299.5482, -82.4563) -> (302.5482, -82.4468)
  line L698 (302.5482, -82.4468) -> (302.5729, -90.192)
  line L699 (302.5729, -90.192) -> (299.5728, -90.2012)
  line L700 (299.5728, -90.2012) -> (299.5972, -97.8247)
  line L701 (299.5972, -97.8247) -> (302.5972, -97.8148)
  line L702 (302.5972, -97.8148) -> (302.6219, -105.5604)
  line L703 (302.6219, -105.5604) -> (299.6219, -105.5699)
  line L704 (299.6219, -105.5699) -> (299.6462, -113.1927)
  line L705 (299.6462, -113.1927) -> (302.6462, -113.1835)
  line L706 (302.6462, -113.1835) -> (302.6709, -120.9284)
  line L707 (302.6709, -120.9284) -> (299.6709, -120.9379)
  line L708 (299.6709, -120.9379) -> (299.6953, -128.5614)
  line L709 (299.6953, -128.5614) -> (302.6953, -128.5515)
  line L710 (302.6953, -128.5515) -> (302.72, -136.2968)
  line L711 (302.72, -136.2968) -> (299.7203, -136.3063)
  line L712 (299.7203, -136.3063) -> (299.7443, -143.9294)
  line L713 (299.7443, -143.9294) -> (302.7443, -143.9199)
  line L714 (302.7443, -143.9199) -> (302.7694, -151.6651)
  line L715 (302.7694, -151.6651) -> (299.7693, -151.6747)
  line L716 (299.7693, -151.6747) -> (299.7937, -159.2978)
  line L717 (299.7937, -159.2978) -> (302.7933, -159.2883)
  line L718 (302.7933, -159.2883) -> (302.8184, -167.0332)
  line L719 (302.8184, -167.0332) -> (299.8184, -167.043)
  line L720 (299.8184, -167.043) -> (299.8279, -170.043)
  line L721 (299.8279, -170.043) -> (291.1002, -170.0709)
  line L722 (291.1002, -170.0709) -> (291.0907, -167.0709)
  line L723 (291.0907, -167.0709) -> (282.4854, -167.0984)
  line L724 (282.4854, -167.0984) -> (282.4949, -170.0984)
  line L725 (282.4949, -170.0984) -> (273.7669, -170.1263)
  line L726 (595.7569, -652.1727) -> (595.7993, -659.8565)
  line L727 (595.7993, -659.8565) -> (598.7993, -659.8399)
  line L728 (598.7993, -659.8399) -> (598.8416, -667.5851)
  line L729 (598.8416, -667.5851) -> (595.8419, -667.6017)
  line L730 (595.8419, -667.6017) -> (595.8839, -675.2245)
  line L731 (595.8839, -675.2245) -> (598.8836, -675.2079)
  line L732 (598.8836, -675.2079) -> (598.9263, -682.9535)
  line L733 (598.9263, -682.9535) -> (595.9263, -682.9694)
  line L734 (595.9263, -682.9694) -> (595.9682, -690.5929)
  line L735 (595.9682, -690.5929) -> (598.9682, -690.5763)
  line L736 (598.9682, -690.5763) -> (599.0109, -698.3212)
  line L737 (599.0109, -698.3212) -> (596.0109, -698.3377)
  line L738 (596.0109, -698.3377) -> (596.0533, -705.9609)
  line L739 (596.0533, -705.9609) -> (599.0529, -705.9443)
  line L740 (599.0529, -705.9443) -> (599.096, -713.6895)
  line L741 (599.096, -713.6895) -> (596.0959, -713.7058)
  line L742 (596.0959, -713.7058) -> (596.1379, -721.3293)
  line L743 (596.1379, -721.3293) -> (599.1379, -721.3127)
  line L744 (599.1379, -721.3127) -> (599.1803, -729.0576)
  line L745 (599.1803, -729.0576) -> (596.1806, -729.0741)
  line L746 (596.1806, -729.0741) -> (596.2226, -736.6973)
  line L747 (596.2226, -736.6973) -> (599.2222, -736.6807)
  line L748 (599.2222, -736.6807) -> (599.2649, -744.4256)
  line L749 (599.2649, -744.4256) -> (596.2649, -744.4422)
  line L750 (596.2649, -744.4422) -> (596.3069, -752.0657)
  line L751 (596.3069, -752.0657) -> (599.3069, -752.0491)
  line L752 (599.3069, -752.0491) -> (599.3496, -759.7939)
  line L753 (599.3496, -759.7939) -> (596.3496, -759.8105)
  line L754 (596.3496, -759.8105) -> (596.3916, -767.4337)
  line L755 (596.3916, -767.4337) -> (599.3916, -767.4171)
  line L756 (599.3916, -767.4171) -> (599.4343, -775.162)
  line L757 (599.4343, -775.162) -> (596.4346, -775.1785)
  line L758 (596.4346, -775.1785) -> (596.4766, -782.8017)
  line L759 (596.4766, -782.8017) -> (599.4766, -782.7851)
  line L760 (599.4766, -782.7851) -> (599.5193, -790.5303)
  line L761 (599.5193, -790.5303) -> (596.5193, -790.5469)
  line L762 (596.5193, -790.5469) -> (596.5616, -798.2308)
  line L763 (596.5616, -798.2308) -> (596.5613, -798.1697)
  line L764 (596.5613, -798.1697) -> (599.5609, -798.1531)
  line L765 (599.5609, -798.1531) -> (599.5613, -798.2142)
  line L766 (599.5613, -798.2142) -> (599.5778, -801.2142)
  line L767 (599.5778, -801.2142) -> (596.5778, -801.2304)
  line L768 (596.5778, -801.2304) -> (587.9133, -801.2787)
  line L769 (587.9133, -801.2787) -> (587.8967, -798.2787)
  line L770 (587.8967, -798.2787) -> (579.3542, -798.3256)
  line L771 (579.3542, -798.3256) -> (579.3704, -801.3253)
  line L772 (579.3704, -801.3253) -> (570.7062, -801.3733)
  line L773 (570.7062, -801.3733) -> (570.6897, -798.3729)
  line L774 (570.6897, -798.3729) -> (562.1468, -798.4202)
  line L775 (562.1468, -798.4202) -> (562.1634, -801.4199)
  line L776 (562.1634, -801.4199) -> (553.4988, -801.4682)
  line L777 (553.4988, -801.4682) -> (553.4823, -798.4682)
  line L778 (553.4823, -798.4682) -> (544.9398, -798.5154)
  line L779 (544.9398, -798.5154) -> (544.9563, -801.5155)
  line L780 (544.9563, -801.5155) -> (536.2914, -801.5627)
  line L781 (536.2914, -801.5627) -> (536.2749, -798.5624)
  line L782 (536.2749, -798.5624) -> (527.7324, -798.61)
  line L783 (527.7324, -798.61) -> (527.7489, -801.6096)
  line L784 (527.7489, -801.6096) -> (519.0844, -801.6576)
  line L785 (519.0844, -801.6576) -> (519.0678, -798.6576)
  line L786 (519.0678, -798.6576) -> (510.5253, -798.7049)
  line L787 (510.5253, -798.7049) -> (510.5419, -801.7045)
  line L788 (510.5419, -801.7045) -> (501.877, -801.7525)
  line L789 (501.877, -801.7525) -> (501.8608, -798.7525)
  line L790 (501.8608, -798.7525) -> (493.3179, -798.7994)
  line L791 (493.3179, -798.7994) -> (493.3345, -801.7991)
  line L792 (493.3345, -801.7991) -> (484.6699, -801.8474)
  line L793 (484.6699, -801.8474) -> (484.6534, -798.8474)
  line L794 (484.6534, -798.8474) -> (476.1105, -798.8943)
  line L795 (476.1105, -798.8943) -> (476.1271, -801.894)
  line L796 (476.1271, -801.894) -> (467.4629, -801.9423)
  line L797 (467.4629, -801.9423) -> (467.4463, -798.9423)
  line L798 (467.4463, -798.9423) -> (458.9035, -798.9889)
  line L799 (458.9035, -798.9889) -> (458.9201, -801.9885)
  line L800 (458.9201, -801.9885) -> (450.2551, -802.0369)
  line L801 (450.2551, -802.0369) -> (450.2389, -799.0368)
  line L802 (450.2389, -799.0368) -> (441.6964, -799.0841)
  line L803 (441.6964, -799.0841) -> (441.713, -802.0841)
  line L804 (441.713, -802.0841) -> (433.0481, -802.1318)
  line L805 (433.0481, -802.1318) -> (433.0315, -799.1314)
  line L806 (433.0315, -799.1314) -> (424.489, -799.179)
  line L807 (424.489, -799.179) -> (424.5056, -802.1783)
  line L808 (424.5056, -802.1783) -> (415.8411, -802.2263)
  line L809 (415.8411, -802.2263) -> (415.8245, -799.2263)
  line L810 (415.8245, -799.2263) -> (407.2816, -799.2736)
  line L811 (407.2816, -799.2736) -> (407.2982, -802.2736)
  line L812 (407.2982, -802.2736) -> (398.6337, -802.3212)
  line L813 (398.6337, -802.3212) -> (398.6171, -799.3208)
  line L814 (398.6171, -799.3208) -> (390.0746, -799.3685)
  line L815 (390.0746, -799.3685) -> (390.0908, -802.3681)
  line L816 (390.0908, -802.3681) -> (381.4266, -802.4161)
  line L817 (381.4266, -802.4161) -> (381.41, -799.4161)
  line L818 (381.41, -799.4161) -> (372.8672, -799.463)
  line L819 (372.8672, -799.463) -> (372.8838, -802.463)
  line L820 (372.8838, -802.463) -> (364.2192, -802.511)
  line L821 (364.2192, -802.511) -> (364.2026, -799.511)
  line L822 (364.2026, -799.511) -> (355.6598, -799.5579)
  line L823 (355.6598, -799.5579) -> (355.6764, -802.5576)
  line L824 (355.6764, -802.5576) -> (347.0118, -802.6055)
  line L825 (347.0118, -802.6055) -> (346.9956, -799.6055)
  line L826 (346.9956, -799.6055) -> (338.4527, -799.6528)
  line L827 (338.4527, -799.6528) -> (338.4693, -802.6528)
  line L828 (338.4693, -802.6528) -> (329.8048, -802.7004)
  line L829 (329.8048, -802.7004) -> (329.7878, -799.7001)
  line L830 (329.7878, -799.7001) -> (321.2457, -799.7477)
  line L831 (321.2457, -799.7477) -> (321.2623, -802.7474)
  line L832 (321.2623, -802.7474) -> (312.597, -802.7953)
  line L833 (312.597, -802.7953) -> (312.5811, -799.7953)
  line L834 (312.5811, -799.7953) -> (304.0383, -799.8422)
  line L835 (304.0383, -799.8422) -> (304.0549, -802.8423)
  line L836 (304.0549, -802.8423) -> (295.3903, -802.8899)
  line L837 (295.3903, -802.8899) -> (295.3734, -799.8899)
  line L838 (295.3734, -799.8899) -> (286.8309, -799.9371)
  line L839 (286.8309, -799.9371) -> (286.8475, -802.9368)
  line L840 (286.8475, -802.9368) -> (278.1829, -802.9851)
  line L841 (278.1829, -802.9851) -> (278.1663, -799.9851)
  line L842 (278.1663, -799.9851) -> (269.6239, -800.032)
  line L843 (269.6239, -800.032) -> (269.6404, -803.0313)
  line L844 (269.6404, -803.0313) -> (260.9759, -803.0797)
  line L845 (260.9759, -803.0797) -> (260.9593, -800.0797)
  line L846 (260.9593, -800.0797) -> (252.4165, -800.1266)
  line L847 (252.4165, -800.1266) -> (252.433, -803.1262)
  line L848 (252.433, -803.1262) -> (243.7685, -803.1746)
  line L849 (243.7685, -803.1746) -> (243.7519, -800.1746)
  line L850 (243.7519, -800.1746) -> (235.2094, -800.2218)
  line L851 (235.2094, -800.2218) -> (235.226, -803.2215)
  line L852 (235.226, -803.2215) -> (226.5614, -803.2691)
  line L853 (226.5614, -803.2691) -> (226.5449, -800.2687)
  line L854 (226.5449, -800.2687) -> (218.002, -800.3164)
  line L855 (218.002, -800.3164) -> (218.0186, -803.316)
  line L856 (218.0186, -803.316) -> (209.354, -803.364)
  line L857 (209.354, -803.364) -> (209.3371, -800.3636)
  line L858 (209.3371, -800.3636) -> (200.795, -800.4113)
  line L859 (200.795, -800.4113) -> (200.8112, -803.4113)